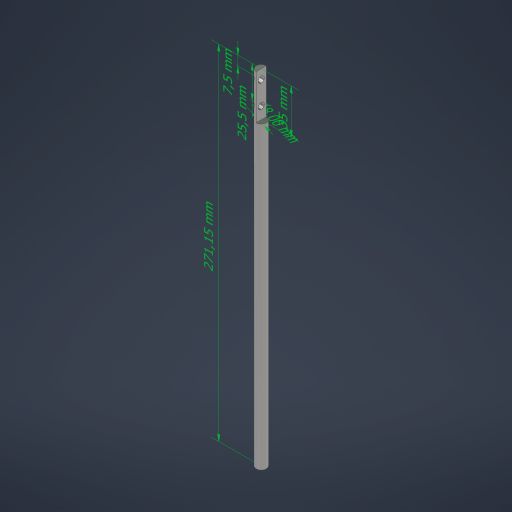
# Autodesk Inventor part: bar
Saved by Autodesk Inventor 2023 (Build 270158000, 158)
## iProperties
Created: 2022-04-23
Part Number: bar
Material: Stainless Steel
Document SubType Name: Modeling
Designer: Norbert Ligas
Density: 8 g/cm^3
Appearance: Semi-Polished
Mass: 100.809 g
Surface Area: 67.8666 cm^2
Volume: 12.6011 cm^3
bar_length: 271,147
pipe_length: 271,147 mm
bar_connection: 35,000 mm
pipe_connection: 35,000 mm
Author: Norbert Ligas
Autodesk Inventor part; units mm, degrees
ref_plane "YZ Plane" through (0, 0, 0) normal (1, 0, 0) x (0, 1, 0)
ref_plane "XZ Plane" through (0, 0, 0) normal (0, 1, 0) x (-1, 0, 0)
ref_plane "XY Plane" through (0, 0, 0) normal (0, 0, 1) x (1, 0, 0)
sketch "Sketch1" plane through (0, 0, 0) normal (0, 1, 0) x (-1, 0, 0)
  circle A0 centre (0, 0) radius 4
  dimension "d0" = 8
  constraints: 1 centre point, 1 coincident
  measures "d0" diameter of A0
extrude "Extrusion1" add sketch "Sketch1" along normal blind 271.1467
sketch "Sketch2" plane through (0, 0, 0) normal (1, 0, 0) x (0, 1, 0)
  line L0 (-54.2293, 0) -> (325.3761, 0) projected
  line L1 (271.1467, -4) -> (271.1467, 4) projected
  line L2 (0, 4) -> (271.1467, 4) projected
  line L3 (271.1467, -4) -> (236.1467, -4)
  line L4 (236.1467, -4) -> (236.1467, 4)
  line L5 (236.1467, 4) -> (271.1467, 4)
  line L6 (271.1467, 4) -> (271.1467, -4)
  point P0 (0, 0)
  point P1 (263.6467, 0)
  point P2 (245.6467, 0)
  dimension "d4" = 7.5
  dimension "d5" = 18
  dimension "d6" = 35
  constraints: 8 end point, 3 point on line, 2 parallel, 1 horizontal, 1 perpendicular
  measures "d4" distance from line of L1 point (263.647, 0)
  measures "d5" distance of point (245.647, 0) point (263.647, 0)
  measures "d6" distance between parallel lines of L1 L4
extrude "Extrusion2" cut sketch "Sketch2" along normal blind 5
hole "Hole1" at (0, 263.6467, 0) at (0, 245.6467, 0) direction (-1, 0, 0) diameter 5 end through all
body "Solid1"
